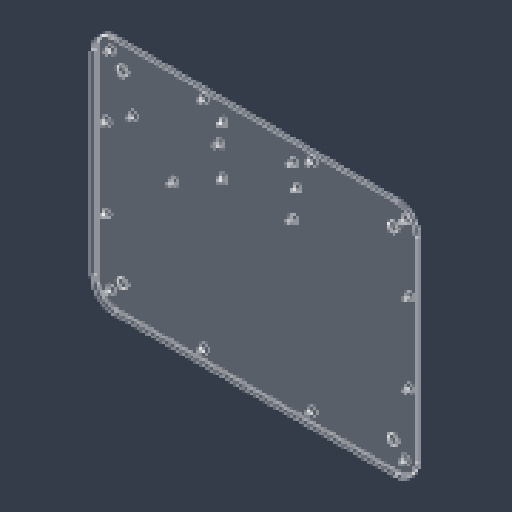
# Autodesk Inventor part: Bottom Plate Sanwa
Saved by Autodesk Inventor 2023.4 (Build 274418000, 418)
## iProperties
Created: 2024-02-20
Part Number: Bottom Plate Sanwa
Material: Polycarbonate, Clear
Document SubType Name: Modeling
Designer: JoaoSilva
Density: 1.2 g/cm^3
Appearance: Polycarbonate - Clear
Author: JoaoSilva
Autodesk Inventor part; units mm, degrees
ref_plane "YZ Plane" through (0, 0, 0) normal (1, 0, 0) x (0, 1, 0)
ref_plane "XZ Plane" through (0, 0, 0) normal (0, 1, 0) x (-1, 0, 0)
ref_plane "XY Plane" through (0, 0, 0) normal (0, 0, 1) x (1, 0, 0)
sketch "Sketch1" plane through (0, 0, 0) normal (0, 0, 1) x (1, 0, 0)
  line L0 (-150, 110) -> (150, 110)
  line L1 (150, 110) -> (150, -110)
  line L2 (150, -110) -> (-150, -110)
  line L3 (-150, -110) -> (-150, 110)
  line L4 (-150, 110) -> (150, -110) construction
  line L5 (150, 110) -> (-150, -110) construction
  point P0 (0, 0)
  dimension "d0" = 300
  dimension "d1" = 220
  constraints: 12 end point, 2 midpoint, 2 parallel, 1 horizontal, 1 perpendicular
  measures "d0" distance of L0.start L0.end
  measures "d1" distance of L2.end L0.start
extrude "Extrusion1" add sketch "Sketch1" along normal blind 5
fillet "Fillet2" radius 20 4 edges at (-150, 110, 2.5) (-150, -110, 2.5) (150, -110, 2.5) (150, 110, 2.5)
chamfer "Chamfer1" distance 1 angle 45 8 edges at (0, -110, 0) (144.1421, -104.1421, 0) (150, 0, 0) (144.1421, 104.1421, 0) (0, 110, 0) (-144.1421, 104.1421, 0) (-150, 0, 0) (-144.1421, -104.1421, 0)
sketch "Sketch8" plane through (0, 0, 0) normal (0, 0, 1) x (1, 0, 0)
  line L0 (-130, 110) -> (130, 110) projected
  line L1 (-150, -90) -> (-150, 90) projected
  point P0 (0, 0)
  point P1 (-140, 37)
  point P2 (-50, 100)
  point P3 (-136, 96)
  dimension "d100" = 14
  dimension "d101" = 14
  dimension "d102" = 10
  dimension "d103" = 10
  dimension "d104" = 100
  dimension "d105" = 73
  measures "d100" distance from line of L0 point (-136, 96)
  measures "d101" distance from line of point (-136, 96) L1
  measures "d102" distance from line of L0 point (-50, 100)
  measures "d103" distance from line of L1 point (-140, 37)
  measures "d104" distance from line of L1 point (-50, 100)
  measures "d105" distance from line of L0 point (-140, 37)
hole "Hole4" at (-140, 37, 0) at (-50, 100, 0) at (-136, 96, 0) direction (0, 0, 1) diameter 3.4 end through all countersink diameter 7.5 countersink angle 90 clearance for "Countersunk Flat Head Hex Socket Screw ISO 10642" size "M3" standard "ISO"
mirror "Mirror1" about plane through (0, 0, 0) normal (1, 0, 0) of "Hole4"
mirror "Mirror2" about plane through (0, 0, 0) normal (0, 1, 0) of "Hole4", "Mirror1"
sketch "Sketch9" plane through (0, 0, 0) normal (0, 0, -1) x (-1, 0, 0)
  line L0 (125, -85) -> (-125, -85) construction
  line L1 (-125, -85) -> (-125, 85) construction
  line L2 (-125, 85) -> (125, 85) construction
  line L3 (125, 85) -> (125, -85) construction
  line L4 (150, 90) -> (150, -90) projected
  line L5 (-130, 110) -> (130, 110) projected
  point P0 (0, 0)
  point P1 (0, 85)
  point P2 (-125, 0)
  dimension "d106" = 25
  dimension "d107" = 25
  constraints: 8 end point, 2 midpoint, 2 parallel, 1 horizontal, 1 horizontal alignment, 1 perpendicular, 1 vertical alignment
  measures "d106" distance between parallel lines of L4 L3
  measures "d107" distance between parallel lines of L5 L2
hole "Hole5" at (-125, -85, 0) at (125, 85, 0) at (125, -85, 0) at (-125, 85, 0) direction (0, 0, 1) diameter 9 depth 2
sketch "Sketch10" plane through (0, 0, 0) normal (0, 0, -1) x (-1, 0, 0)
  line L0 (-35.7, 71.2) -> (35.7, 71.2) construction
  point P0 (0, 71.2)
  point P1 (0, 0)
  dimension "d115" = 71.2
  dimension "d116" = 71.4
  constraints: 2 end point, 1 horizontal, 1 midpoint, 1 vertical alignment
  measures "d115" distance from line of point (0, 0) L0
  measures "d116" distance of L0.start L0.end
hole "Hole6" at (35.7, 71.2, 0) at (-35.7, 71.2, 0) direction (0, 0, 1) diameter 3.4 end through all countersink diameter 7.5 countersink angle 90 clearance for "Countersunk Flat Head Hex Socket Screw ISO 10642" size "M3" standard "ISO"
sketch "Sketch11" plane through (0, 0, 0) normal (0, 0, -1) x (-1, 0, 0)
  line L0 (77.9535, 19.5226) -> (115.4377, 53.3631) construction
  line L1 (34.4702, 98.6683) -> (96.6956, 36.4429) construction
  line L2 (-130, 110) -> (130, 110) projected
  point P0 (0, 0)
  dimension "d124" = 50.5
  dimension "d134" = 87.076
  dimension "d135" = 88
  dimension "d136" = 45
  constraints: 4 end point, 1 midpoint, 1 other
  measures "d124" distance of L0.start L0.end
  measures "d134" angle of L1 L0
  measures "d135" distance of L1.start L1.end
  measures "d136" angle of L2 L1
hole "Hole7" at (-77.9535, 19.5226, 0) at (-115.4377, 53.3631, 0) direction (0, 0, 1) diameter 3.4 end through all countersink diameter 7.5 countersink angle 90 clearance for "Countersunk Flat Head Hex Socket Screw ISO 10642" size "M3" standard "ISO"
sketch "Sketch12" plane through (0, 0, 0) normal (0, 0, -1) x (-1, 0, 0)
  line L0 (-32.5, 90) -> (32.5, 90) construction
  line L1 (32.5, 90) -> (32.5, 45) construction
  line L2 (32.5, 45) -> (-32.5, 45) construction
  line L3 (-32.5, 45) -> (-32.5, 90) construction
  point P0 (0, 0)
  point P1 (0, 45)
  dimension "d137" = 45
  dimension "d138" = 45
  dimension "d139" = 65
  constraints: 8 end point, 2 parallel, 1 horizontal, 1 midpoint, 1 perpendicular, 1 vertical alignment
  measures "d137" distance from line of point (0, 0) L2
  measures "d138" distance of L0.end L1.end
  measures "d139" distance of L1.end L2.end
hole "Hole8" at (32.5, 90, 0) at (-32.5, 45, 0) at (-32.5, 90, 0) at (32.5, 45, 0) direction (0, 0, 1) diameter 3.4 end through all countersink diameter 7.5 countersink angle 90 clearance for "Countersunk Flat Head Hex Socket Screw ISO 10642" size "M3" standard "ISO"
equation "\"d101\" = d100"
equation "\"d103\" = d102"
equation "\"d107\" = d106"
body "Solid1"
